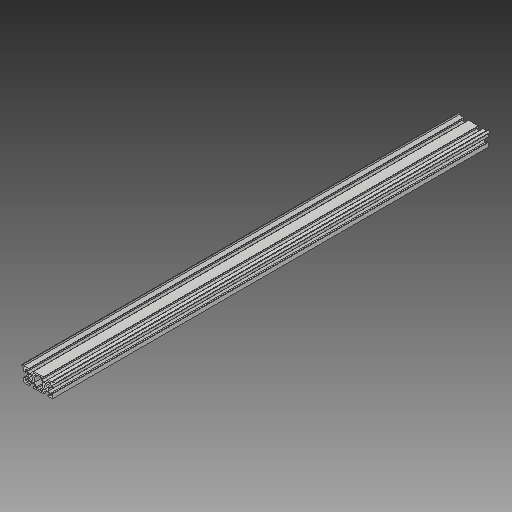
# Autodesk Inventor part: Makerslide 600mm
Saved by Autodesk Inventor 2018 (Build 220112000, 112)
## iProperties
Created: 2016-07-11
Part Number: Makerslide 600mm
Material: Generic
Document SubType Name: Modeling
Designer: joshm
Density: 1 g/cm^3
Appearance: Default
Author: joshm
Autodesk Inventor part; units mm, degrees
ref_plane "YZ Plane" through (0, 0, 0) normal (1, 0, 0) x (0, 1, 0)
ref_plane "XZ Plane" through (0, 0, 0) normal (0, 1, 0) x (-1, 0, 0)
ref_plane "XY Plane" through (0, 0, 0) normal (0, 0, 1) x (1, 0, 0)
sketch "Sketch1" plane through (0, 0, 0) normal (0, 0, 1) x (1, 0, 0)
  line L0 (-2.5, 7.3119) -> (2.5, 7.3119) projected
  line L1 (2.5, 7.3119) -> (2.5, 5.7513) projected
  line L2 (2.5, 5.7513) -> (6, 2.2513) projected
  line L3 (6, 2.2513) -> (6, -3.6274) projected
  line L4 (6, -3.6274) -> (2.5, -7.1274) projected
  line L5 (2.5, -7.1274) -> (2.5, -8.6881) projected
  line L6 (2.5, -8.6881) -> (-2.5, -8.6881) projected
  line L7 (-2.5, -8.6881) -> (-2.5, -7.1274) projected
  line L8 (-2.5, -7.1274) -> (-6, -3.6274) projected
  line L9 (-6, -3.6274) -> (-6, 2.2513) projected
  line L10 (-6, 2.2513) -> (-2.5, 5.7513) projected
  line L11 (-2.5, 5.7513) -> (-2.5, 7.3119) projected
  circle A0 centre (10, -0.6881) radius 2.1 projected
  circle A1 centre (-10, -0.6881) radius 2.1 projected
  line L12 (-4, 6.3726) -> (-7.0607, 3.3119) projected
  line L13 (-7.0607, 3.3119) -> (-9.7, 3.3119) projected
  line L14 (-9.7, 3.3119) -> (-10, 3.0119) projected
  line L15 (-10, 3.0119) -> (-10.3, 3.3119) projected
  line L16 (-10.3, 3.3119) -> (-12.9393, 3.3119) projected
  line L17 (-12.9393, 3.3119) -> (-16, 6.3726) projected
  line L18 (-16, 6.3726) -> (-16, 7.3119) projected
  line L19 (-16, 7.3119) -> (-13, 7.3119) projected
  line L20 (-13, 7.3119) -> (-13, 9.0119) projected
  arc A2 (-13, 9.0119) -> (-13.3, 9.3119) centre (-13.3, 9.0119) ccw projected
  line L21 (-13.3, 9.3119) -> (-20, 9.3119) projected
  line L22 (-20, 9.3119) -> (-20, 11.6869) projected
  line L23 (-20, 11.6869) -> (-20.5929, 11.6869) projected
  arc A3 (-20.5929, 11.6869) -> (-20.9464, 11.5405) centre (-20.5929, 11.1869) ccw projected
  line L24 (-20.9464, 11.5405) -> (-22.8214, 9.6655) projected
  arc A4 (-22.8214, 9.6655) -> (-22.8214, 8.9584) centre (-22.4679, 9.3119) ccw projected
  line L25 (-22.8214, 8.9584) -> (-20.9464, 7.0834) projected
  arc A5 (-20.9464, 7.0834) -> (-20.5929, 6.9369) centre (-20.5929, 7.4369) ccw projected
  line L26 (-20.5929, 6.9369) -> (-20.5, 6.9369) projected
  arc A6 (-20, 6.4369) -> (-20.5, 6.9369) centre (-20.5, 6.4369) ccw projected
  line L27 (-20, 6.4369) -> (-20, 2.6119) projected
  arc A7 (-20, 2.6119) -> (-19.7, 2.3119) centre (-19.7, 2.6119) ccw projected
  line L28 (-19.7, 2.3119) -> (-18, 2.3119) projected
  line L29 (-18, 2.3119) -> (-18, 5.3119) projected
  line L30 (-18, 5.3119) -> (-17.0607, 5.3119) projected
  line L31 (-17.0607, 5.3119) -> (-14, 2.2513) projected
  line L32 (-14, 2.2513) -> (-14, -0.3881) projected
  line L33 (-14, -0.3881) -> (-13.7, -0.6881) projected
  line L34 (-13.7, -0.6881) -> (-14, -0.9881) projected
  line L35 (-14, -0.9881) -> (-14, -3.6274) projected
  line L36 (-14, -3.6274) -> (-17.0607, -6.6881) projected
  line L37 (-17.0607, -6.6881) -> (-18, -6.6881) projected
  line L38 (-18, -6.6881) -> (-18, -3.6881) projected
  line L39 (-18, -3.6881) -> (-19.7, -3.6881) projected
  arc A8 (-19.7, -3.6881) -> (-20, -3.9881) centre (-19.7, -3.9881) ccw projected
  line L40 (-20, -3.9881) -> (-20, -9.6881) projected
  arc A9 (-20, -9.6881) -> (-19, -10.6881) centre (-19, -9.6881) ccw projected
  line L41 (-19, -10.6881) -> (-13.3, -10.6881) projected
  arc A10 (-13.3, -10.6881) -> (-13, -10.3881) centre (-13.3, -10.3881) ccw projected
  line L42 (-13, -10.3881) -> (-13, -8.6881) projected
  line L43 (-13, -8.6881) -> (-16, -8.6881) projected
  line L44 (-16, -8.6881) -> (-16, -7.7487) projected
  line L45 (-16, -7.7487) -> (-12.9393, -4.6881) projected
  line L46 (-12.9393, -4.6881) -> (-10.3, -4.6881) projected
  line L47 (-10.3, -4.6881) -> (-10, -4.3881) projected
  line L48 (-10, -4.3881) -> (-9.7, -4.6881) projected
  line L49 (-9.7, -4.6881) -> (-7.0607, -4.6881) projected
  line L50 (-7.0607, -4.6881) -> (-4, -7.7487) projected
  line L51 (-4, -7.7487) -> (-4, -8.6881) projected
  line L52 (-4, -8.6881) -> (-7, -8.6881) projected
  line L53 (-7, -8.6881) -> (-7, -10.3881) projected
  arc A11 (-7, -10.3881) -> (-6.7, -10.6881) centre (-6.7, -10.3881) ccw projected
  line L54 (-6.7, -10.6881) -> (6.7, -10.6881) projected
  arc A12 (6.7, -10.6881) -> (7, -10.3881) centre (6.7, -10.3881) ccw projected
  line L55 (7, -10.3881) -> (7, -8.6881) projected
  line L56 (7, -8.6881) -> (4, -8.6881) projected
  line L57 (4, -8.6881) -> (4, -7.7487) projected
  line L58 (4, -7.7487) -> (7.0607, -4.6881) projected
  line L59 (7.0607, -4.6881) -> (9.7, -4.6881) projected
  line L60 (9.7, -4.6881) -> (10, -4.3881) projected
  line L61 (10, -4.3881) -> (10.3, -4.6881) projected
  line L62 (10.3, -4.6881) -> (12.9393, -4.6881) projected
  line L63 (12.9393, -4.6881) -> (16, -7.7487) projected
  line L64 (16, -7.7487) -> (16, -8.6881) projected
  line L65 (16, -8.6881) -> (13, -8.6881) projected
  line L66 (13, -8.6881) -> (13, -10.3881) projected
  arc A13 (13, -10.3881) -> (13.3, -10.6881) centre (13.3, -10.3881) ccw projected
  line L67 (13.3, -10.6881) -> (19, -10.6881) projected
  arc A14 (19, -10.6881) -> (20, -9.6881) centre (19, -9.6881) ccw projected
  line L68 (20, -9.6881) -> (20, -3.9881) projected
  arc A15 (20, -3.9881) -> (19.7, -3.6881) centre (19.7, -3.9881) ccw projected
  line L69 (19.7, -3.6881) -> (18, -3.6881) projected
  line L70 (18, -3.6881) -> (18, -6.6881) projected
  line L71 (18, -6.6881) -> (17.0607, -6.6881) projected
  line L72 (17.0607, -6.6881) -> (14, -3.6274) projected
  line L73 (14, -3.6274) -> (14, -0.9881) projected
  line L74 (14, -0.9881) -> (13.7, -0.6881) projected
  line L75 (13.7, -0.6881) -> (14, -0.3881) projected
  line L76 (14, -0.3881) -> (14, 2.2513) projected
  line L77 (14, 2.2513) -> (17.0607, 5.3119) projected
  line L78 (17.0607, 5.3119) -> (18, 5.3119) projected
  line L79 (18, 5.3119) -> (18, 2.3119) projected
  line L80 (18, 2.3119) -> (19.7, 2.3119) projected
  arc A16 (19.7, 2.3119) -> (20, 2.6119) centre (19.7, 2.6119) ccw projected
  line L81 (20, 2.6119) -> (20, 6.4369) projected
  arc A17 (20.5, 6.9369) -> (20, 6.4369) centre (20.5, 6.4369) ccw projected
  line L82 (20.5, 6.9369) -> (20.5929, 6.9369) projected
  arc A18 (20.5929, 6.9369) -> (20.9464, 7.0834) centre (20.5929, 7.4369) ccw projected
  line L83 (20.9464, 7.0834) -> (22.8214, 8.9584) projected
  arc A19 (22.8214, 8.9584) -> (22.8214, 9.6655) centre (22.4679, 9.3119) ccw projected
  line L84 (22.8214, 9.6655) -> (20.9464, 11.5405) projected
  arc A20 (20.9464, 11.5405) -> (20.5929, 11.6869) centre (20.5929, 11.1869) ccw projected
  line L85 (20.5929, 11.6869) -> (20, 11.6869) projected
  line L86 (20, 11.6869) -> (20, 9.3119) projected
  line L87 (20, 9.3119) -> (13.3, 9.3119) projected
  arc A21 (13.3, 9.3119) -> (13, 9.0119) centre (13.3, 9.0119) ccw projected
  line L88 (13, 9.0119) -> (13, 7.3119) projected
  line L89 (13, 7.3119) -> (16, 7.3119) projected
  line L90 (16, 7.3119) -> (16, 6.3726) projected
  line L91 (16, 6.3726) -> (12.9393, 3.3119) projected
  line L92 (12.9393, 3.3119) -> (10.3, 3.3119) projected
  line L93 (10.3, 3.3119) -> (10, 3.0119) projected
  line L94 (10, 3.0119) -> (9.7, 3.3119) projected
  line L95 (9.7, 3.3119) -> (7.0607, 3.3119) projected
  line L96 (7.0607, 3.3119) -> (4, 6.3726) projected
  line L97 (4, 6.3726) -> (4, 7.3119) projected
  line L98 (4, 7.3119) -> (7, 7.3119) projected
  line L99 (7, 7.3119) -> (7, 9.0119) projected
  arc A22 (7, 9.0119) -> (6.7, 9.3119) centre (6.7, 9.0119) ccw projected
  line L100 (6.7, 9.3119) -> (-6.7, 9.3119) projected
  arc A23 (-6.7, 9.3119) -> (-7, 9.0119) centre (-6.7, 9.0119) ccw projected
  line L101 (-7, 9.0119) -> (-7, 7.3119) projected
  line L102 (-7, 7.3119) -> (-4, 7.3119) projected
  line L103 (-4, 7.3119) -> (-4, 6.3726) projected
  point P0 (0, 0)
extrude "Extrusion1" add sketch "Sketch1" along normal blind 600
body "Solid1"
